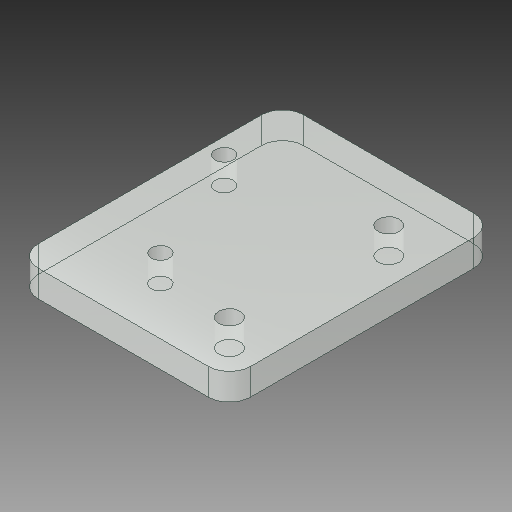
# Autodesk Inventor part: Soporte_Final_Carrera
Saved by Autodesk Inventor 2019 (Build 230136000, 136)
## iProperties
Created: 2020-04-05
Part Number: Soporte_Final_Carrera
Material: Generic
Document SubType Name: Modeling
Designer: Jurgen
Density: 1 g/cm^3
Appearance: Clear
Mass: 9.71487 g
Surface Area: 49.8409 cm^2
Volume: 9.71487 cm^3
Author: Jurgen
Autodesk Inventor part; units mm, degrees
ref_plane "YZ Plane" through (0, 0, 0) normal (1, 0, 0) x (0, 1, 0)
ref_plane "XZ Plane" through (0, 0, 0) normal (0, 1, 0) x (-1, 0, 0)
ref_plane "XY Plane" through (0, 0, 0) normal (0, 0, 1) x (1, 0, 0)
sketch "Sketch1" plane through (0, 0, 0) normal (0, 1, 0) x (-1, 0, 0)
  line L0 (-20, 25) -> (20, 25)
  line L1 (20, 25) -> (20, -25)
  line L2 (20, -25) -> (-20, -25)
  line L3 (-20, -25) -> (-20, 25)
  line L4 (-20, 25) -> (20, -25) construction
  line L5 (20, 25) -> (-20, -25) construction
  line L6 (17, 14) -> (7, 14) construction
  arc A0 (7, 14) -> (4, 11) centre (7, 11) ccw construction
  line L7 (4, 11) -> (4, -11) construction
  arc A1 (4, -11) -> (7, -14) centre (7, -11) ccw construction
  line L8 (7, -14) -> (17, -14) construction
  arc A2 (17, -14) -> (20, -11) centre (17, -11) ccw construction
  line L9 (20, -11) -> (20, 11) construction
  arc A3 (20, 11) -> (17, 14) centre (17, 11) ccw construction
  circle A4 centre (17.5, -0.5) radius 2 construction
  circle A5 centre (17, 11) radius 1.7 construction
  circle A6 centre (7, -11) radius 1.7 construction
  line L10 (4, 0) -> (20, 0) construction
  line L11 (17, -14) -> (7, -14) construction
  arc A7 (4, -11) -> (7, -14) centre (7, -11) ccw construction
  line L12 (4, -11) -> (4, 11) construction
  arc A8 (7, 14) -> (4, 11) centre (7, 11) ccw construction
  line L13 (7, 14) -> (17, 14) construction
  arc A9 (20, 11) -> (17, 14) centre (17, 11) ccw construction
  line L14 (20, 11) -> (20, -11) construction
  arc A10 (17, -14) -> (20, -11) centre (17, -11) ccw construction
  circle A11 centre (17.5, 0.5) radius 2 construction
  circle A12 centre (17, -11) radius 1.7
  circle A13 centre (7, 11) radius 1.7
  line L15 (20, 0) -> (-20, 0) construction
  line L16 (0, 25) -> (0, -25) construction
  line L17 (-10, 25) -> (-10, -25) construction
  circle A14 centre (-10, 15) radius 2
  circle A15 centre (-10, -15) radius 2
  point P0 (0, 0)
  point P1 (12, 0)
  dimension "d0" = 40
  dimension "d1" = 50
  dimension "d5" = 10
  dimension "d6" = 4
  dimension "d7" = 4
  dimension "d8" = 10
  dimension "d9" = 10
  constraints: 36 end point, 16 centre point, 16 point on circle, 15 symmetric about line, 8 midpoint, 4 point on line, 2 parallel, 2 perpendicular, 1 horizontal, 7 other
  measures "d0" distance of L1.end L2.end
  measures "d1" distance of L0.end L1.end
  measures "d5" distance between parallel lines of L3 L17
  measures "d6" diameter of A14
  measures "d7" diameter of A15
  measures "d8" distance from line of L0 A14.centre
  measures "d9" distance from line of L2 A15.centre
extrude "Extrusion2" add sketch "Sketch1" along normal blind 5
fillet "Fillet2" radius 4 4 edges at (20, 2.5, -25) (20, 2.5, 25) (-20, 2.5, -25) (-20, 2.5, 25)
body "Solid2"
